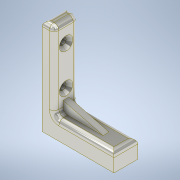
# Autodesk Inventor part: LightLBracket
Saved by Autodesk Inventor 2021.2 (Build 252289000, 289)
## iProperties
Created: 2021-02-27
Part Number: LightLBracket
Material: PC/ABS Plastic
Document SubType Name: Modeling
Designer: robst
Density: 0.357273 g/cm^3
Appearance: Silver
Author: robst
Autodesk Inventor part; units mm, degrees
ref_plane "YZ Plane" through (0, 0, 0) normal (1, 0, 0) x (0, 1, 0)
ref_plane "XZ Plane" through (0, 0, 0) normal (0, 1, 0) x (-1, 0, 0)
ref_plane "XY Plane" through (0, 0, 0) normal (0, 0, 1) x (1, 0, 0)
sketch "Sketch1" plane through (0, 0, 0) normal (0, 0, 1) x (1, 0, 0)
  line L0 (0, 0) -> (-38.1, 0)
  line L1 (-38.1, 0) -> (-38.1, 9.525)
  line L2 (-38.1, 9.525) -> (-6.35, 9.525)
  line L3 (-6.35, 9.525) -> (-6.35, 50.8)
  line L4 (-6.35, 50.8) -> (0, 50.8)
  line L5 (0, 50.8) -> (0, 0)
  dimension "d0" = 38.1
  dimension "d1" = 9.525
  dimension "d2" = 50.8
  dimension "d3" = 6.35
  constraints: 12 end point, 5 perpendicular, 1 horizontal
  measures "d0" distance from line of L1 L0.start
  measures "d1" distance between parallel lines of L2 L0
  measures "d2" distance from line of L4 L0.start
  measures "d3" distance between parallel lines of L5 L3
extrude "Extrusion1" add sketch "Sketch1" along normal mid plane 12.7
sketch "Sketch2" plane through (-6.35, 9.525, 6.35) normal (-1, 0, 0) x (0, 0, 1)
  line L0 (-12.7, 41.275) -> (0, 41.275) construction
  line L1 (-6.35, 41.275) -> (-6.35, 0) construction
  line L2 (-12.7, 0) -> (0, 0) construction
  point P0 (-6.35, -9.525)
  point P1 (-6.35, 30.9563)
  point P2 (-6.35, 10.3188)
  dimension "d6" = 10.3187
  dimension "d7" = 10.3187
  constraints: 2 end point, 2 midpoint, 2 point on line
  measures "d6" distance from line of point (-6.35, 30.956) L0
  measures "d7" distance from line of point (-6.35, 10.319) L2
hole "Hole1" at (-6.35, 40.4812, 0) at (-6.35, 19.8438, 0) direction (1, 0, 0) diameter 3.81 end through all countersink diameter 7.0866 countersink angle 82 clearance for "Flat Head Machine Screw (82)" size "#6" standard "Ansi Unified Screw Threads"
sketch "Sketch3" plane through (-38.1, 0, 6.35) normal (0, -1, 0) x (1, 0, 0)
  line L0 (38.1, -6.35) -> (0, -6.35) construction
  line L1 (0, -12.7) -> (0, 0) construction
  line L2 (38.1, -12.7) -> (38.1, 0) projected
  point P0 (7.62, -6.35)
  dimension "d15" = 30.48
  constraints: 2 end point, 1 midpoint, 1 point on line
  measures "d15" distance from line of point (7.62, -6.35) L2
hole "Hole2" at (-30.48, 0, 0) direction (0, 1, 0) diameter 3.302 depth 8.89 thread size "8-32 UNC" class "2B" standard "ANSI Unified Screw Threads"
fillet "FilletForTop" radius 2.54 4 edges at (-6.35, 50.8, 0) (-3.175, 50.8, 6.35) (0, 50.8, 0) (-3.175, 50.8, -6.35)
fillet "FilletForFront" radius 2.54 8 edges at (-5.6061, 50.0561, -5.6061) (-6.35, 28.8925, -6.35) (-5.6061, 50.0561, 5.6061) (-6.35, 28.8925, 6.35) (-6.35, 9.525, 0) (-38.1, 9.525, 0) (-22.225, 9.525, 6.35) (-22.225, 9.525, -6.35)
sketch "Sketch4" plane through (0, 0, 0) normal (0, 0, 1) x (1, 0, 0)
  line L0 (-6.35, 48.26) -> (-6.35, 12.065) projected
  line L1 (-8.89, 9.525) -> (-35.56, 9.525) projected
  line L2 (-6.35, 15.0304) -> (-27.559, 9.525)
  line L3 (-4.4654, 17.9387) -> (-6.35, 16.3004) projected
  line L4 (-28.829, 8.89) -> (-28.829, 0) projected
  line L5 (-6.35, 15.0304) -> (-6.35, 9.525)
  line L6 (-6.35, 9.525) -> (-27.559, 9.525)
  point P0 (0, 0)
  point P1 (-6.35, 12.065)
  dimension "d26" = 1.27
  dimension "d27" = 1.27
  constraints: 6 end point, 2 point on line, 1 collinear, 1 vertical
  measures "d26" distance of L3.end L2.start
  measures "d27" distance from line of L2.end L4
extrude "Extrusion2" add sketch "Sketch4" along normal mid plane 3.175
equation "\"d0\" = distanceFromWall"
equation "\"d1\" = baseThickness"
equation "\"d2\" = wallHeight"
equation "\"d3\" = wallThickness"
equation "\"d4\" = width"
equation "\"d6\" = wallHoleCentersDistanceFromEnd"
equation "\"d7\" = wallHoleCentersDistanceFromEnd"
equation "\"d15\" = lightHoleDistanceFromWall"
equation "\"d28\" = 0.25 * width"
equation "\"baseThickness\" = 9.525"
equation "\"wallThickness\" = 6.35"
equation "\"distanceFromWall\" = 38.1"
equation "\"wallHeight\" = 50.8"
equation "\"width\" = 12.7"
equation "\"baseHeight\" = wallHeight - baseThickness"
equation "\"wallHoleCentersDistanceFromEnd\" = 0.25 * baseHeight"
equation "\"lightHoleDistanceFromWall\" = 30.48"
equation "\"screwDepth\" = 7.62"
body "Solid1"
